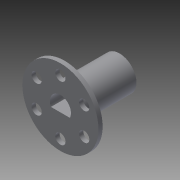
# Autodesk Inventor part: axe_roue_moteur
Saved by Autodesk Inventor 2014 SP1 (Build 180222100, 222)
## iProperties
Created: 2014-09-07
Part Number: axe_roue_moteur
Material: Générique
Document SubType Name: Modeling
Designer: astralien3000
Density: 1 g/cm^3
Appearance: Par défaut
Author: astralien3000
Autodesk Inventor part; units mm, degrees
ref_plane "YZ Plane" through (0, 0, 0) normal (1, 0, 0) x (0, 1, 0)
ref_plane "XZ Plane" through (0, 0, 0) normal (0, 1, 0) x (-1, 0, 0)
ref_plane "XY Plane" through (0, 0, 0) normal (0, 0, 1) x (1, 0, 0)
sketch "Esquisse1" plane through (0, 0, 0) normal (0, 1, 0) x (-1, 0, 0)
  circle A0 centre (0, 0) radius 9
  dimension "d0" = 18
  constraints: 1 centre point, 1 coincident
  measures "d0" diameter of A0
extrude "Extrusion1" add sketch "Esquisse1" along normal blind 1
sketch "Esquisse2" plane through (0, 1, 0) normal (0, 1, 0) x (1, 0, 0)
  circle A0 centre (0, 0) radius 9 projected
  circle A1 centre (0, 0) radius 4
  dimension "d3" = 8
  constraints: 1 centre point, 1 coincident
  measures "d3" diameter of A1
extrude "Extrusion2" add sketch "Esquisse2" along normal blind 13 contours A1
sketch "Esquisse3" plane through (0, 14, 0) normal (0, 1, 0) x (1, 0, 0)
  circle A0 centre (0, 0) radius 4 projected
  arc A1 (-2.25, 1.0897) -> (2.25, 1.0897) centre (0, 0) ccw
  line L0 (-2.25, 1.0897) -> (2.25, 1.0897)
  arc A2 (2.25, 1.0897) -> (-2.25, 1.0897) centre (0, 0) ccw
  dimension "d6" = 5
  dimension "d10" = 4.5
  constraints: 4 point on circle, 2 centre point, 2 end point, 1 coincident, 1 horizontal
  measures "d6" diameter of A1
  measures "d10" distance of L0.start L0.end
extrude "Extrusion3" cut sketch "Esquisse3" against normal through all contours L0 A1
sketch "Esquisse4" plane through (-2.25, 14, -1.0897) normal (0, 0, 1) x (1, 0, 0)
  line L0 (0, 0) -> (4.5, 0) projected
  line L1 (2.25, -14) -> (2.25, 0) construction
  circle A0 centre (2.25, -10) radius 1.5
  dimension "d11" = 4
  dimension "d12" = 3
  constraints: 2 end point, 1 centre point, 1 midpoint, 1 point on line
  measures "d11" distance of L1.start A0.centre
  measures "d12" diameter of A0
extrude "Extrusion4" cut sketch "Esquisse4" against normal up to next
sketch "Esquisse5" plane through (0, 1, 0) normal (0, 1, 0) x (1, 0, 0)
  circle A0 centre (0, 0) radius 4 projected
  circle A1 centre (0, 0) radius 9 projected
  line L0 (0, 0) -> (0, 9) construction
  circle A2 centre (0, 6.5) radius 1.2128
  dimension "d15" = 2.4255
  dimension "d16" = 6.5
  constraints: 2 end point, 1 centre point, 1 point on line, 1 vertical, 1 vertical alignment, 1 other
  measures "d15" diameter of A2
  measures "d16" distance of A0.centre A2.centre
extrude "Extrusion5" cut sketch "Esquisse5" against normal up to next contours A2
pattern_circular "Réseau circulaire1" count 6 over 360 about axis through (0, -10, 0) along (0, 1, 0) of "Extrusion5"
thread "Filetage1" size "M3x0.5" class "6H" standard "ANSI Metric M Profile" full length
